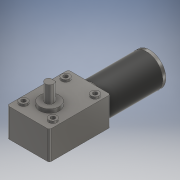
# Autodesk Inventor part: TS-40GZ495
Saved by Autodesk Inventor 2017 (Build 210142000, 142)
## iProperties
Created: 2019-11-11
Part Number: TS-40GZ495
Material: Stainless Steel
Document SubType Name: Modeling
Designer: Dell
Density: 8 g/cm^3
Appearance: Semi-Polished
Author: Dell
Autodesk Inventor part; units mm, degrees
ref_plane "YZ Plane" through (0, 0, 0) normal (1, 0, 0) x (0, 1, 0)
ref_plane "XZ Plane" through (0, 0, 0) normal (0, 1, 0) x (-1, 0, 0)
ref_plane "XY Plane" through (0, 0, 0) normal (0, 0, 1) x (1, 0, 0)
sketch "Sketch1" plane through (0, 0, 0) normal (0, 0, 1) x (1, 0, 0)
  line L0 (0, 0) -> (40.12, 0)
  line L1 (40.12, 0) -> (40.12, 58.1)
  line L2 (40.12, 58.1) -> (0, 58.1)
  line L3 (0, 58.1) -> (0, 0)
  circle A0 centre (20.06, 20.2) radius 4
  line L4 (6.06, 49.5) -> (34.06, 49.5) construction
  line L5 (34.06, 49.5) -> (34.06, 9.5) construction
  line L6 (34.06, 9.5) -> (6.06, 9.5) construction
  line L7 (6.06, 9.5) -> (6.06, 49.5) construction
  circle A1 centre (6.06, 49.5) radius 2
  circle A2 centre (34.06, 49.5) radius 2
  circle A3 centre (34.06, 9.5) radius 2
  circle A4 centre (6.06, 9.5) radius 2
  point P0 (20.06, 58.1)
  point P1 (20.06, 49.5)
  dimension "d0" = 40.12
  dimension "d1" = 58.1
  dimension "d2" = 8
  dimension "d3" = 37.9
  dimension "d4" = 28
  dimension "d5" = 40
  dimension "d6" = 8.6
  dimension "d7" = 4
  dimension "d8" = 4
  dimension "d9" = 4
  dimension "d10" = 4
  constraints: 16 end point, 5 centre point, 4 coincident, 4 parallel, 2 horizontal, 2 midpoint, 2 perpendicular, 2 vertical alignment
  measures "d0" distance of L2.end L1.end
  measures "d1" distance of L1.end L0.end
  measures "d2" diameter of A0
  measures "d3" distance from line of A0.centre L2
  measures "d4" distance of L4.start L4.end
  measures "d5" distance of L6.end L4.start
  measures "d6" distance between parallel lines of L2 L4
  measures "d7" diameter of A1
  measures "d8" diameter of A2
  measures "d9" diameter of A3
  measures "d10" diameter of A4
extrude "Extrusion1" add sketch "Sketch1" along normal blind 27
sketch "Sketch2" plane through (0, 0, 27) normal (0, 0, 1) x (1, 0, 0)
  circle A0 centre (6.06, 49.5) radius 2 projected
  circle A1 centre (34.06, 49.5) radius 2 projected
  circle A2 centre (20.06, 20.2) radius 4 projected
  circle A3 centre (34.06, 9.5) radius 2 projected
  circle A4 centre (6.06, 9.5) radius 2 projected
  circle A5 centre (6.06, 49.5) radius 2 projected
  circle A6 centre (6.06, 49.5) radius 3.9
  circle A7 centre (34.06, 9.5) radius 2 projected
  circle A8 centre (34.06, 9.5) radius 3.9
  circle A9 centre (34.06, 49.5) radius 2 projected
  circle A10 centre (34.06, 49.5) radius 3.9
  circle A11 centre (6.06, 9.5) radius 3.9
  circle A12 centre (20.06, 20.2) radius 9.375
  point P0 (0, 0)
  dimension "d13" = 7.8
  dimension "d14" = 7.8
  dimension "d15" = 7.8
  dimension "d16" = 7.8
  dimension "d17" = 18.75
  constraints: 5 centre point, 5 coincident
  measures "d13" diameter of A6
  measures "d14" diameter of A10
  measures "d15" diameter of A8
  measures "d16" diameter of A11
  measures "d17" diameter of A12
extrude "Extrusion2" add sketch "Sketch2" along normal blind 2
sketch "Sketch3" plane through (0, 0, 27) normal (0, 0, 1) x (1, 0, 0)
  circle A0 centre (20.06, 20.2) radius 9.375 projected
  circle A1 centre (20.06, 20.2) radius 4 projected
  point P0 (0, 0)
extrude "Extrusion3" add sketch "Sketch3" along normal blind 3.5
sketch "Sketch4" plane through (0, 0, 0) normal (0, 0, -1) x (-1, 0, 0)
  circle A0 centre (-20.06, 20.2) radius 9.375 projected
  circle A1 centre (-20.06, 20.2) radius 4 projected
  point P0 (0, 0)
extrude "Extrusion4" add sketch "Sketch4" along normal blind 3.5
sketch "Sketch5" plane through (20.06, 20.2, -3.5) normal (0, 0, -1) x (-1, 0, 0)
  circle A0 centre (0, 0) radius 9.375 projected
  point P0 (20.06, -20.2)
extrude "Extrusion5" add sketch "Sketch5" against normal up to surface (34 mm away) from surface at 0
sketch "Sketch6" plane through (20.06, 20.2, 30.5) normal (0, 0, 1) x (1, 0, 0)
  circle A0 centre (0, 0) radius 4
  circle A1 centre (0, 0) radius 9.375 projected
  point P0 (-20.06, -20.2)
  dimension "d26" = 8
  constraints: 1 centre point, 1 coincident
  measures "d26" diameter of A0
extrude "Extrusion6" add sketch "Sketch6" along normal blind 16 contours A0
sketch "Sketch7" plane through (20.06, 20.2, 46.5) normal (0, 0, 1) x (1, 0, 0)
  line L0 (-2.6458, 3) -> (2.6458, 3)
  circle A0 centre (0, 0) radius 4 projected
  arc A1 (-2.6458, 3) -> (2.6458, 3) centre (0, 0) ccw
  point P0 (-20.06, -20.2)
  point P1 (0, 3)
  dimension "d29" = 7
  constraints: 2 end point, 2 point on circle, 1 centre point, 1 horizontal, 1 midpoint, 1 vertical alignment, 3 other
extrude "Extrusion7" cut sketch "Sketch7" against normal blind 13 contours A0 L0 picked at (0.5822, 3.4764)
sketch "Sketch8" plane through (0, 58.1, 0) normal (0, 1, 0) x (1, 0, 0)
  circle A0 centre (20.06, -9.5) radius 15.5
  line L0 (40.12, -27) -> (0, -27) projected
  line L1 (40.12, 0) -> (40.12, -27) projected
  line L2 (40.12, -13.5) -> (0, -13.5)
  point P0 (0, 0)
  point P1 (20.06, -27)
  point P2 (20.06, -13.5)
  dimension "d32" = 31
  dimension "d34" = 4
  constraints: 3 midpoint, 2 end point, 2 vertical alignment, 1 centre point, 1 horizontal
  measures "d32" diameter of A0
  measures "d34" distance of point (20.06, -13.5) A0.centre
extrude "Extrusion8" add sketch "Sketch8" along normal blind 57.2
sketch "Sketch10" plane through (20.06, 115.3, 9.5) normal (0, 1, 0) x (1, 0, 0)
  circle A0 centre (0, 0) radius 6
  circle A1 centre (0, 0) radius 15.5 projected
  point P0 (-20.06, 9.5)
  dimension "d37" = 12
  constraints: 1 centre point, 1 coincident
  measures "d37" diameter of A0
extrude "Extrusion9" add sketch "Sketch10" along normal blind 2 contours A0
sketch "Sketch11" plane through (20.06, 115.3, 9.5) normal (0, 1, 0) x (1, 0, 0)
  circle A0 centre (0, 0) radius 15.5 projected
  circle A1 centre (0, 0) radius 15.4
  point P0 (-20.06, 9.5)
  dimension "d40" = 0.1
  constraints: 1 centre point
  measures "d40" radial gap between concentric circles of A0 A1
extrude "Extrusion10" cut sketch "Sketch11" against normal blind 3
sketch "Sketch12" plane through (0, 58.1, 27) normal (0, 1, 0) x (1, 0, 0)
  circle A0 centre (20.06, 17.5) radius 15.4 projected
  circle A1 centre (20.06, 17.5) radius 15.5 projected
  point P0 (0, 27)
extrude "Extrusion11" cut sketch "Sketch12" along normal blind 3
sketch "Sketch13" plane through (0, 0, 0) normal (0, 0, -1) x (-1, 0, 0)
  circle A0 centre (-6.06, 49.5) radius 3.9 projected
  circle A1 centre (-34.06, 49.5) radius 3.9 projected
  circle A2 centre (-34.06, 9.5) radius 3.9 projected
  circle A3 centre (-6.06, 9.5) radius 3.9 projected
  circle A4 centre (-6.06, 9.5) radius 2 projected
  circle A5 centre (-6.06, 49.5) radius 2 projected
  circle A6 centre (-34.06, 49.5) radius 2 projected
  circle A7 centre (-34.06, 9.5) radius 2 projected
  point P0 (0, 0)
extrude "Extrusion12" add sketch "Sketch13" along normal blind 2
fillet "Fillet1" radius 2 4 edges at (40.12, 58.1, 13.5) (0, 58.1, 13.5) (0, 0, 13.5) (40.12, 0, 13.5)
body "Solid1"
